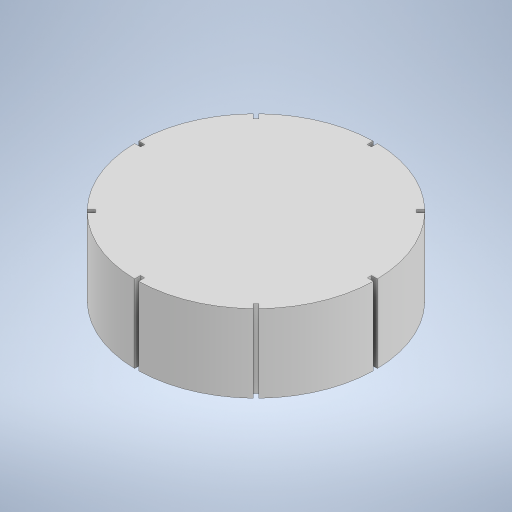
# Autodesk Inventor part: 屋-2 柱-1
Saved by Autodesk Inventor 2024 (Build 280153000, 153)
## iProperties
Created: 2024-05-21
Part Number: 屋-2 柱-1
Material: 一般
Document SubType Name: Modeling
Designer: User
Density: 1 g/cm^3
Appearance: 預設
Author: User
Autodesk Inventor part; units mm, degrees
ref_plane "YZ Plane" through (0, 0, 0) normal (1, 0, 0) x (0, 1, 0)
ref_plane "XZ Plane" through (0, 0, 0) normal (0, 1, 0) x (-1, 0, 0)
ref_plane "XY Plane" through (0, 0, 0) normal (0, 0, 1) x (1, 0, 0)
sketch "草圖1" plane through (0, 0, 0) normal (0, 1, 0) x (-1, 0, 0)
  circle A0 centre (0, 0) radius 20
  dimension "d0" = 40
  constraints: 1 centre point, 1 coincident
  measures "d0" diameter of A0
extrude "擠出1" add sketch "草圖1" along normal blind 13
sketch "草圖2" plane through (0, 13, 0) normal (0, 1, 0) x (1, 0, 0)
  circle A0 centre (0, 0) radius 19
  circle A1 centre (0, 0) radius 20 projected
  line L0 (-20, 0) -> (-19, 0)
  line L1 (0, 0) -> (-19.997, 0.349)
  line L2 (0, 0) -> (-19.997, -0.349)
  line L3 (0, 0) -> (-14.3868, -13.8932)
  line L4 (0, 0) -> (-13.8932, -14.3868)
  line L5 (0, 0) -> (-0.349, -19.997)
  line L6 (0, 0) -> (0.349, -19.997)
  line L7 (0, 0) -> (13.8932, -14.3868)
  line L8 (0, 0) -> (14.3868, -13.8932)
  line L9 (0, 0) -> (19.997, -0.349)
  line L10 (0, 0) -> (19.997, 0.349)
  line L11 (0, 0) -> (14.3868, 13.8932)
  line L12 (0, 0) -> (13.8932, 14.3868)
  line L13 (0, 0) -> (0.349, 19.997)
  line L14 (0, 0) -> (-0.349, 19.997)
  line L15 (0, 0) -> (-13.8932, 14.3868)
  line L16 (0, 0) -> (-14.3868, 13.8932)
  point P0 (13.1985, 13.6675)
  point P1 (13.6675, 13.1985)
  point P2 (18.9971, 0.3316)
  point P3 (18.9971, -0.3316)
  point P4 (13.6675, -13.1985)
  point P5 (13.1985, -13.6675)
  point P6 (0.3316, -18.9971)
  point P7 (-0.3316, -18.9971)
  point P8 (-13.1985, -13.6675)
  point P9 (-13.6675, -13.1985)
  point P10 (-18.9971, -0.3316)
  point P11 (-18.9971, 0.3316)
  point P12 (-13.6675, 13.1985)
  point P13 (-13.1985, 13.6675)
  point P14 (-0.3316, 18.9971)
  point P15 (0.3316, 18.9971)
  dimension "d3" = 38
  dimension "d6" = 1
  dimension "d7" = 1
  dimension "d10" = 360
  constraints: 34 end point, 3 coincident, 3 point on circle, 2 horizontal, 42 other
  measures "d6" angle of L1 L0
  measures "d7" angle of L2 L0
extrude "擠出2" cut sketch "草圖2" against normal up to next contours A0 L10 A1 L9 | A0 L12 A1 L11 | L8 A1 L7 A0 | A0 L0 A1 L1 | L2 A1 L0 A0 | A0 L4 A1 L3 | A0 L6 A1 L5 | A0 L14 A1 L13 | A0 L16 A1 L15
